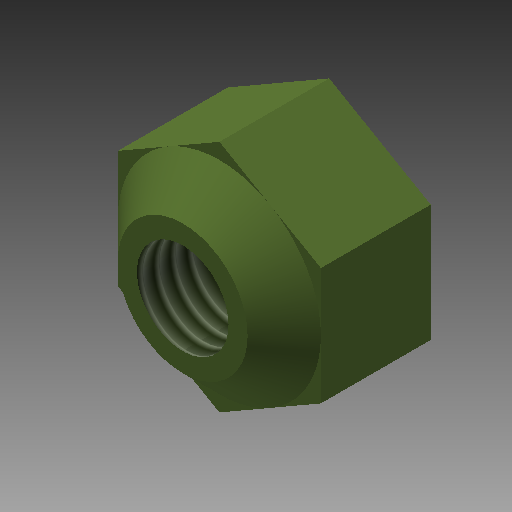
# Autodesk Inventor part: ナイロンナット
Saved by Autodesk Inventor 2017.3 (Build 213256000, 256)
## iProperties
Created: 2016-03-12
Part Number: ナイロンナット
Material: アルミニウム
Document SubType Name: Modeling
Designer: 大空
Density: 2.7 g/cm^3
Appearance: オリーブ グリーン
Mass: 0.206945 g
Surface Area: 1.38318 cm^2
Volume: 0.0766463 cm^3
Author: 大空
Autodesk Inventor part; units mm, degrees
ref_plane "YZ Plane" through (0, 0, 0) normal (1, 0, 0) x (0, 1, 0)
ref_plane "XZ Plane" through (0, 0, 0) normal (0, 1, 0) x (-1, 0, 0)
ref_plane "XY Plane" through (0, 0, 0) normal (0, 0, 1) x (1, 0, 0)
sketch "スケッチ1" plane through (0, 0, 0) normal (0, 0, 1) x (1, 0, 0)
  line L0 (0, -3.2) -> (-2.7713, -1.6)
  line L1 (-2.7713, -1.6) -> (-2.7713, 1.6)
  line L2 (-2.7713, 1.6) -> (0, 3.2)
  line L3 (0, 3.2) -> (2.7713, 1.6)
  line L4 (2.7713, 1.6) -> (2.7713, -1.6)
  line L5 (2.7713, -1.6) -> (0, -3.2)
  circle A0 centre (0, 0) radius 2.7713
  dimension "d0" = 6.4
  constraints: 12 end point, 2 coincident, 1 centre point, 13 other
  measures "d0" distance of L0.start L2.end
extrude "押し出し1" add sketch "スケッチ1" along normal blind 3
sketch "スケッチ2" plane through (0, 0, 3) normal (0, 0, 1) x (1, 0, 0)
  line L0 (-2.7713, -1.6) -> (0, -3.2) projected
  line L1 (0, -3.2) -> (2.7713, -1.6) projected
  line L2 (2.7713, -1.6) -> (2.7713, 1.6) projected
  line L3 (2.7713, 1.6) -> (0, 3.2) projected
  line L4 (0, 3.2) -> (-2.7713, 1.6) projected
  line L5 (-2.7713, 1.6) -> (-2.7713, -1.6) projected
  circle A0 centre (0, 0) radius 2.7713
  constraints: 1 centre point, 1 coincident, 1 tangent
extrude "押し出し2" add sketch "スケッチ2" along normal blind 1 contours A0
chamfer "面取り1" distance 1 angle 45 1 edges at (-2.7713, 0, 4)
sketch "スケッチ3" plane through (0, 0, 4) normal (0, 0, 1) x (1, 0, 0)
  circle A0 centre (0, 0) radius 1.7713 projected
  circle A1 centre (0, 0) radius 1.25
  dimension "d8" = 2.5
  constraints: 1 centre point, 1 coincident
  measures "d8" diameter of A1
extrude "押し出し3" cut sketch "スケッチ3" against normal blind 4 contours A1
thread "ねじ1" size "M2.5x0.45" class "6H" standard "ANSI Metric M Profile" full length
